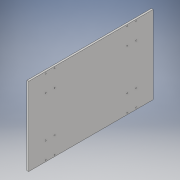
# Autodesk Inventor part: PlateFrame
Saved by Autodesk Inventor 2017 (Build 210142000, 142)
## iProperties
Created: 2017-09-27
Part Number: PlateFrame
Material: Generic
Document SubType Name: Modeling
Designer: User
Density: 1 g/cm^3
Appearance: Default
Author: User
Autodesk Inventor part; units mm, degrees
ref_plane "YZ Plane" through (0, 0, 0) normal (1, 0, 0) x (0, 1, 0)
ref_plane "XZ Plane" through (0, 0, 0) normal (0, 1, 0) x (-1, 0, 0)
ref_plane "XY Plane" through (0, 0, 0) normal (0, 0, 1) x (1, 0, 0)
sketch "Sketch1" plane through (0, 0, 0) normal (1, 0, 0) x (0, 1, 0)
  line L0 (0, 0) -> (279.4, 0)
  line L1 (279.4, 0) -> (279.4, -444.5)
  line L2 (279.4, -444.5) -> (0, -444.5)
  line L3 (0, -444.5) -> (0, 0)
  circle A0 centre (273.4056, -60.198) radius 1.9431
  circle A1 centre (273.4056, -92.202) radius 1.9431
  circle A2 centre (213.36, -60.198) radius 1.9431
  circle A3 centre (213.36, -92.202) radius 1.9431
  circle A4 centre (66.04, -60.198) radius 1.9431
  circle A5 centre (66.04, -92.202) radius 1.9431
  circle A6 centre (5.9944, -60.198) radius 1.9431
  circle A7 centre (5.9944, -92.202) radius 1.9431
  circle A8 centre (273.4056, -352.298) radius 1.9431
  circle A9 centre (273.4056, -384.302) radius 1.9431
  circle A10 centre (213.36, -352.298) radius 1.9431
  circle A11 centre (213.36, -384.302) radius 1.9431
  circle A12 centre (66.04, -352.298) radius 1.9431
  circle A13 centre (66.04, -384.302) radius 1.9431
  circle A14 centre (5.9944, -384.302) radius 1.9431
  circle A15 centre (5.9944, -352.298) radius 1.9431
  dimension "d0" = 279.4
  dimension "d1" = 444.5
  dimension "d2" = 3.8862
  dimension "d3" = 3.8862
  dimension "d4" = 32.004
  dimension "d5" = 5.9944
  dimension "d6" = 5.9944
  dimension "d7" = 60.198
  dimension "d8" = 3.8862
  dimension "d9" = 3.8862
  dimension "d10" = 60.0456
  dimension "d11" = 60.0456
  dimension "d12" = 60.198
  dimension "d13" = 3.8862
  dimension "d14" = 3.8862
  dimension "d15" = 3.8862
  dimension "d16" = 3.8862
  dimension "d17" = 60.198
  dimension "d18" = 60.198
  dimension "d19" = 5.9944
  dimension "d20" = 5.9944
  dimension "d22" = 60.0456
  dimension "d23" = 60.0456
  dimension "d24" = 32.004
  dimension "d25" = 3.8862
  dimension "d26" = 3.8862
  dimension "d27" = 5.9944
  dimension "d28" = 5.9944
  dimension "d29" = 3.8862
  dimension "d30" = 3.8862
  dimension "d32" = 32.004
  dimension "d33" = 32.004
  dimension "d34" = 60.198
  dimension "d35" = 60.198
  dimension "d36" = 3.8862
  dimension "d37" = 3.8862
  dimension "d38" = 3.8862
  dimension "d39" = 3.8862
  constraints: 16 centre point, 8 end point, 2 parallel, 1 horizontal, 1 perpendicular
  measures "d0" distance of L1.end L2.end
  measures "d1" distance of L0.end L1.end
  measures "d2" diameter of A0
  measures "d3" diameter of A1
  measures "d4" distance of A1.centre A0.centre
  measures "d5" distance from line of L1 A0.centre
  measures "d6" distance from line of L1 A1.centre
  measures "d7" distance from line of A0.centre L0
  measures "d8" diameter of A2
  measures "d9" diameter of A3
  measures "d10" distance of A0.centre A2.centre
  measures "d11" distance of A1.centre A3.centre
  measures "d12" distance from line of L0 A2.centre
  measures "d13" diameter of A4
  measures "d14" diameter of A5
  measures "d15" diameter of A6
  measures "d16" diameter of A7
  measures "d17" distance from line of L0 A4.centre
  measures "d18" distance from line of L0 A6.centre
  measures "d19" distance from line of L3 A6.centre
  measures "d20" distance from line of L3 A7.centre
  measures "d22" distance of A6.centre A4.centre
  measures "d23" distance of A5.centre A7.centre
  measures "d24" distance of A5.centre A4.centre
  measures "d25" diameter of A8
  measures "d26" diameter of A9
  measures "d27" distance from line of L1 A8.centre
  measures "d28" distance from line of L1 A9.centre
  measures "d29" diameter of A10
  measures "d30" diameter of A11
  measures "d32" distance of A8.centre A9.centre
  measures "d33" distance of A11.centre A10.centre
  measures "d34" distance from line of L2 A9.centre
  measures "d35" distance from line of L2 A11.centre
  measures "d36" diameter of A12
  measures "d37" diameter of A13
  measures "d38" diameter of A14
  measures "d39" diameter of A15
extrude "Extrusion1" add sketch "Sketch1" along normal blind 6.35
equation "\"d3\" = d2"
equation "\"d6\" = d5"
equation "\"d8\" = d2"
equation "\"d9\" = d2"
equation "\"d11\" = d10"
equation "\"d12\" = d7"
equation "\"d13\" = d2"
equation "\"d14\" = d2"
equation "\"d15\" = d2"
equation "\"d16\" = d2"
equation "\"d17\" = d12"
equation "\"d18\" = d7"
equation "\"d19\" = d5"
equation "\"d20\" = d19"
equation "\"d22\" = d10"
equation "\"d23\" = d22"
equation "\"d25\" = d2"
equation "\"d26\" = d25"
equation "\"d27\" = d5"
equation "\"d28\" = d27"
equation "\"d29\" = d25"
equation "\"d30\" = d25"
equation "\"d32\" = d4"
equation "\"d33\" = d32"
equation "\"d34\" = d7"
equation "\"d35\" = d34"
equation "\"d36\" = d2"
equation "\"d37\" = d2"
equation "\"d38\" = d2"
equation "\"d39\" = d2"
body "Solid1"
